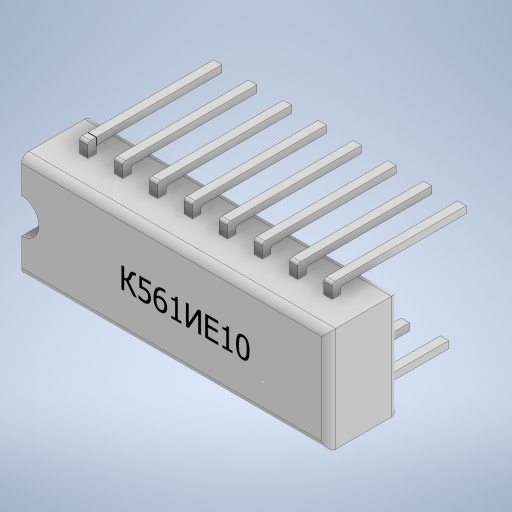
# Autodesk Inventor part: К561ИЕ10
Saved by Autodesk Inventor 2024 (Build 280153000, 153)
## iProperties
Created: 2023-12-20
Part Number: К561ИЕ10
Material: Generic
Document SubType Name: Sheet Metal
Designer: user
Density: 1 g/cm^3
Sheet Metal Rule: Default
Appearance: Default
Author: user
Autodesk Inventor part; units mm, degrees
ref_plane "YZ Plane" through (0, 0, 0) normal (1, 0, 0) x (0, 1, 0)
ref_plane "XZ Plane" through (0, 0, 0) normal (0, 1, 0) x (-1, 0, 0)
sketch "Sketch1" plane through (0, 0, 0) normal (0, 0, 1) x (1, 0, 0)
  line L0 (-17.2939, 5.4021) -> (4.7061, 5.4021)
  line L1 (4.7061, 5.4021) -> (4.7061, -2.0979)
  line L2 (4.7061, -2.0979) -> (-17.2939, -2.0979)
  line L3 (-17.2939, -2.0979) -> (-17.2939, 5.4021)
  line L4 (-17.2939, 5.4021) -> (-17.2939, 2.9021)
  line L5 (-17.2939, 2.9021) -> (-17.2939, 0.4021)
  line L6 (-17.2939, 0.4021) -> (-17.2939, -2.0979)
  arc A0 (-17.2939, 0.4021) -> (-17.2939, 2.9021) centre (-17.3071, 1.6521) ccw
  point P0 (0, 0)
  dimension "d0" = 22
  dimension "d1" = 7.5
  dimension "d2" = 2.5
  dimension "d3" = 2.5
  constraints: 14 end point, 2 parallel, 2 point on circle, 2 point on line, 1 centre point, 1 collinear, 1 horizontal, 1 perpendicular
  measures "d0" distance of L1.end L2.end
  measures "d1" distance of L0.end L1.end
  measures "d2" distance of L0.start L4.end
  measures "d3" distance of L4.end L5.end
extrude "Extrusion1" add sketch "Sketch1" along normal mid plane 5 contours L0 L1 L2 L3 A0
ref_plane "Work Plane1" through (0, 0, 0) normal (0, 0, 1) x (1, 0, 0)
sketch "Sketch2" plane through (0, 0, 0) normal (0, 0, 1) x (1, 0, 0)
  line L0 (4.7061, 5.4021) -> (-17.2939, 5.4021) projected
  line L1 (4.7061, 5.4021) -> (2.4561, 5.4021)
  line L2 (2.4561, 5.4021) -> (-0.0439, 5.4021)
  line L3 (-0.0439, 5.4021) -> (-2.5439, 5.4021)
  line L4 (-2.5439, 5.4021) -> (-5.0439, 5.4021)
  line L5 (-5.0439, 5.4021) -> (-7.5439, 5.4021)
  line L6 (-7.5439, 5.4021) -> (-10.0439, 5.4021)
  line L7 (-10.0439, 5.4021) -> (-12.5439, 5.4021)
  line L8 (-12.5439, 5.4021) -> (-15.0439, 5.4021)
  line L9 (-15.0439, 5.4021) -> (-17.2939, 5.4021)
  point P0 (0, 0)
  dimension "d6" = 2.25
  dimension "d7" = 2.5
  dimension "d8" = 2.5
  dimension "d9" = 2.5
  dimension "d10" = 2.5
  dimension "d11" = 2.5
  dimension "d12" = 2.5
  dimension "d13" = 2.5
  dimension "d14" = 2.25
  constraints: 18 end point, 1 horizontal, 9 other
  measures "d6" distance of L1.start L1.end
  measures "d7" distance of L1.end L2.end
  measures "d8" distance of L2.end L3.end
  measures "d9" distance of L3.end L4.end
  measures "d10" distance of L4.end L5.end
  measures "d11" distance of L5.end L6.end
  measures "d12" distance of L6.end L7.end
  measures "d13" distance of L7.end L8.end
  measures "d14" distance of L8.end L9.end
sketch "Sketch3" plane through (-17.2939, 5.4021, 2.5) normal (0, 1, 0) x (1, 0, 0)
  line L0 (20.1524, 2.9) -> (19.3524, 2.9)
  line L1 (19.3524, 2.9) -> (19.3524, 2.1)
  line L2 (19.3524, 2.1) -> (20.1524, 2.1)
  line L3 (20.1524, 2.1) -> (20.1524, 2.9)
  line L4 (20.1524, 2.9) -> (19.3524, 2.1) construction
  line L5 (19.3524, 2.9) -> (20.1524, 2.1) construction
  line L6 (17.6939, 2.9) -> (16.8939, 2.9)
  line L7 (16.8939, 2.9) -> (16.8939, 2.1)
  line L8 (16.8939, 2.1) -> (17.6939, 2.1)
  line L9 (17.6939, 2.1) -> (17.6939, 2.9)
  line L10 (17.6939, 2.9) -> (16.8939, 2.1) construction
  line L11 (16.8939, 2.9) -> (17.6939, 2.1) construction
  line L12 (15.1521, 2.1) -> (14.3521, 2.1)
  line L13 (14.3521, 2.1) -> (14.3521, 2.9)
  line L14 (14.3521, 2.9) -> (15.1521, 2.9)
  line L15 (15.1521, 2.9) -> (15.1521, 2.1)
  line L16 (15.1521, 2.1) -> (14.3521, 2.9) construction
  line L17 (14.3521, 2.1) -> (15.1521, 2.9) construction
  line L18 (12.6545, 2.1) -> (11.8545, 2.1)
  line L19 (11.8545, 2.1) -> (11.8545, 2.9)
  line L20 (11.8545, 2.9) -> (12.6545, 2.9)
  line L21 (12.6545, 2.9) -> (12.6545, 2.1)
  line L22 (12.6545, 2.1) -> (11.8545, 2.9) construction
  line L23 (11.8545, 2.1) -> (12.6545, 2.9) construction
  line L24 (10.1493, 2.9) -> (9.3493, 2.9)
  line L25 (9.3493, 2.9) -> (9.3493, 2.1)
  line L26 (9.3493, 2.1) -> (10.1493, 2.1)
  line L27 (10.1493, 2.1) -> (10.1493, 2.9)
  line L28 (10.1493, 2.9) -> (9.3493, 2.1) construction
  line L29 (9.3493, 2.9) -> (10.1493, 2.1) construction
  line L30 (7.6538, 2.1) -> (6.8538, 2.1)
  line L31 (6.8538, 2.1) -> (6.8538, 2.9)
  line L32 (6.8538, 2.9) -> (7.6538, 2.9)
  line L33 (7.6538, 2.9) -> (7.6538, 2.1)
  line L34 (7.6538, 2.1) -> (6.8538, 2.9) construction
  line L35 (6.8538, 2.1) -> (7.6538, 2.9) construction
  line L36 (5.1502, 2.1) -> (4.3502, 2.1)
  line L37 (4.3502, 2.1) -> (4.3502, 2.9)
  line L38 (4.3502, 2.9) -> (5.1502, 2.9)
  line L39 (5.1502, 2.9) -> (5.1502, 2.1)
  line L40 (5.1502, 2.1) -> (4.3502, 2.9) construction
  line L41 (4.3502, 2.1) -> (5.1502, 2.9) construction
  line L42 (2.649, 2.1) -> (1.849, 2.1)
  line L43 (1.849, 2.1) -> (1.849, 2.9)
  line L44 (1.849, 2.9) -> (2.649, 2.9)
  line L45 (2.649, 2.9) -> (2.649, 2.1)
  line L46 (2.649, 2.1) -> (1.849, 2.9) construction
  line L47 (1.849, 2.1) -> (2.649, 2.9) construction
  line L48 (20.0524, 2.8) -> (19.4524, 2.8)
  line L49 (19.4524, 2.8) -> (19.4524, 2.2)
  line L50 (19.4524, 2.2) -> (20.0524, 2.2)
  line L51 (20.0524, 2.2) -> (20.0524, 2.8)
  line L52 (20.0524, 2.8) -> (19.4524, 2.2) construction
  line L53 (19.4524, 2.8) -> (20.0524, 2.2) construction
  line L54 (17.5939, 2.8) -> (16.9939, 2.8)
  line L55 (16.9939, 2.8) -> (16.9939, 2.2)
  line L56 (16.9939, 2.2) -> (17.5939, 2.2)
  line L57 (17.5939, 2.2) -> (17.5939, 2.8)
  line L58 (17.5939, 2.8) -> (16.9939, 2.2) construction
  line L59 (16.9939, 2.8) -> (17.5939, 2.2) construction
  line L60 (15.0521, 2.8) -> (14.4521, 2.8)
  line L61 (14.4521, 2.8) -> (14.4521, 2.2)
  line L62 (14.4521, 2.2) -> (15.0521, 2.2)
  line L63 (15.0521, 2.2) -> (15.0521, 2.8)
  line L64 (15.0521, 2.8) -> (14.4521, 2.2) construction
  line L65 (14.4521, 2.8) -> (15.0521, 2.2) construction
  line L66 (12.5545, 2.8) -> (11.9545, 2.8)
  line L67 (11.9545, 2.8) -> (11.9545, 2.2)
  line L68 (11.9545, 2.2) -> (12.5545, 2.2)
  line L69 (12.5545, 2.2) -> (12.5545, 2.8)
  line L70 (12.5545, 2.8) -> (11.9545, 2.2) construction
  line L71 (11.9545, 2.8) -> (12.5545, 2.2) construction
  line L72 (9.4493, 2.8) -> (9.4493, 2.2)
  line L73 (10.0493, 2.2) -> (10.0493, 2.8)
  line L74 (10.0493, 2.8) -> (9.4493, 2.2) construction
  line L75 (9.4493, 2.8) -> (10.0493, 2.2) construction
  line L76 (10.0493, 2.8) -> (9.4493, 2.8)
  line L77 (9.4493, 2.2) -> (10.0493, 2.2)
  line L78 (6.9538, 2.8) -> (6.9538, 2.2)
  line L79 (7.5538, 2.2) -> (7.5538, 2.8)
  line L80 (7.5538, 2.8) -> (6.9538, 2.2) construction
  line L81 (6.9538, 2.8) -> (7.5538, 2.2) construction
  line L82 (7.5538, 2.8) -> (6.9538, 2.8)
  line L83 (6.9538, 2.2) -> (7.5538, 2.2)
  line L84 (4.4502, 2.8) -> (4.4502, 2.2)
  line L85 (5.0502, 2.2) -> (5.0502, 2.8)
  line L86 (5.0502, 2.8) -> (4.4502, 2.2) construction
  line L87 (4.4502, 2.8) -> (5.0502, 2.2) construction
  line L88 (5.0502, 2.8) -> (4.4502, 2.8)
  line L89 (4.4502, 2.2) -> (5.0502, 2.2)
  line L90 (1.949, 2.8) -> (1.949, 2.2)
  line L91 (2.549, 2.2) -> (2.549, 2.8)
  line L92 (2.549, 2.8) -> (1.949, 2.2) construction
  line L93 (1.949, 2.8) -> (2.549, 2.2) construction
  line L94 (2.549, 2.8) -> (1.949, 2.8)
  line L95 (1.949, 2.2) -> (2.549, 2.2)
  point P0 (17.2939, 2.5)
  dimension "d15" = 0.8
  dimension "d16" = 0.8
  dimension "d17" = 0.8
  dimension "d18" = 0.8
  dimension "d19" = 0.8
  dimension "d20" = 0.8
  dimension "d21" = 0.8
  dimension "d22" = 0.8
  dimension "d23" = 0.8
  dimension "d24" = 0.8
  dimension "d25" = 0.8
  dimension "d26" = 0.8
  dimension "d27" = 0.8
  dimension "d28" = 0.8
  dimension "d29" = 0.8
  dimension "d30" = 0.8
  dimension "d31" = 0.6
  dimension "d32" = 0.6
  dimension "d33" = 0.6
  dimension "d34" = 0.6
  dimension "d35" = 0.6
  dimension "d36" = 0.6
  dimension "d37" = 0.6
  dimension "d38" = 0.6
  dimension "d39" = 0.6
  dimension "d40" = 0.6
  dimension "d41" = 0.6
  dimension "d42" = 0.6
  dimension "d43" = 0.6
  dimension "d44" = 0.6
  dimension "d45" = 0.6
  dimension "d46" = 0.6
  constraints: 192 end point, 32 parallel, 16 horizontal, 16 perpendicular, 4 midpoint
  measures "d15" distance of L2.end L1.end
  measures "d16" distance of L1.end L0.end
  measures "d17" distance of L8.end L7.end
  measures "d18" distance of L7.end L6.end
  measures "d19" distance of L13.end L14.end
  measures "d20" distance of L12.end L13.end
  measures "d21" distance of L19.end L20.end
  measures "d22" distance of L18.end L19.end
  measures "d23" distance of L26.end L25.end
  measures "d24" distance of L25.end L24.end
  measures "d25" distance of L32.start L33.start
  measures "d26" distance of L30.end L32.start
  measures "d27" distance of L38.start L39.start
  measures "d28" distance of L36.end L38.start
  measures "d29" distance of L44.start L45.start
  measures "d30" distance of L42.end L44.start
  measures "d31" distance of L50.end L49.end
  measures "d32" distance of L49.end L48.end
  measures "d33" distance of L57.start L55.end
  measures "d34" distance of L55.end L55.start
  measures "d35" distance of L63.start L61.end
  measures "d36" distance of L61.end L61.start
  measures "d37" distance of L69.start L67.end
  measures "d38" distance of L67.end L67.start
  measures "d39" distance of L73.start L72.end
  measures "d40" distance of L72.end L72.start
  measures "d41" distance of L79.start L78.end
  measures "d42" distance of L78.end L78.start
  measures "d43" distance of L85.start L84.end
  measures "d44" distance of L84.end L84.start
  measures "d45" distance of L91.start L90.end
  measures "d46" distance of L90.end L90.start
extrude "Extrusion2" add sketch "Sketch3" along normal blind 1 contours L51 L50 L49 L48 | L57 L56 L55 L54 | L63 L62 L61 L60 | L69 L68 L67 L66 | L76 L73 L77 L72 | L82 L79 L83 L78 | L88 L85 L89 L84 | L94 L91 L95 L90
sketch "Sketch4" plane through (2.7586, 5.4021, -0.3) normal (0, 0, -1) x (-1, 0, 0)
  line L0 (0.6, 0) -> (0.6, 1) projected
  line L1 (0.6, 0.5) -> (0, 0.5)
  line L2 (0, 0) -> (0, 1) projected
  line L3 (2.4586, 0) -> (2.4586, 1) projected
  line L4 (2.4586, 0.5) -> (3.0586, 0.5)
  line L5 (3.0586, 0) -> (3.0586, 1) projected
  line L6 (5.0003, 0) -> (5.0003, 1) projected
  line L7 (5.0003, 0.5) -> (5.6003, 0.5)
  line L8 (5.6003, 0) -> (5.6003, 1) projected
  line L9 (7.4979, 0) -> (7.4979, 1) projected
  line L10 (7.4979, 0.5) -> (8.0979, 0.5)
  line L11 (8.0979, 0) -> (8.0979, 1) projected
  line L12 (10.0031, 0) -> (10.0031, 1) projected
  line L13 (10.0031, 0.5) -> (10.6031, 0.5)
  line L14 (10.6031, 0) -> (10.6031, 1) projected
  line L15 (12.4987, 0) -> (12.4987, 1) projected
  line L16 (12.4987, 0.5) -> (13.0987, 0.5)
  line L17 (13.0987, 0) -> (13.0987, 1) projected
  line L18 (15.0022, 0) -> (15.0022, 1) projected
  line L19 (15.0022, 0.5) -> (15.6022, 0.5)
  line L20 (15.6022, 0) -> (15.6022, 1) projected
  line L21 (17.5034, 0) -> (17.5034, 1) projected
  line L22 (17.5034, 0.5) -> (18.1034, 0.5)
  line L23 (18.1034, 0) -> (18.1034, 1) projected
  line L24 (17.5034, 0.5) -> (17.5034, 1)
  line L25 (17.5034, 1) -> (18.1034, 1)
  line L26 (18.1034, 1) -> (18.1034, 0.5)
  point P0 (2.7586, -5.4021)
  constraints: 22 end point, 16 midpoint, 2 perpendicular
sketch "Sketch5" plane through (2.7586, 5.4021, -0.3) normal (0, 0, -1) x (-1, 0, 0)
  line L0 (0, 0) -> (0, 1) projected
  line L1 (0, 0.5) -> (0, 1)
  line L2 (0.6, 1) -> (0, 1) projected
  line L3 (0, 1) -> (0.6, 1)
  line L4 (0.6, 1) -> (0.6, 0.5)
  line L5 (0.6, 0.5) -> (0, 0.5)
  point P0 (2.7586, -5.4021)
  constraints: 8 end point, 3 perpendicular, 1 collinear, 1 midpoint
sketch "Sketch6" plane through (0.3, 5.4021, -0.3) normal (0, 0, -1) x (-1, 0, 0)
  line L0 (0, 0.5) -> (0, 1)
  line L1 (0, 1) -> (0.6, 1)
  line L2 (0.6, 1) -> (0.6, 0.5)
  line L3 (0.6, 0.5) -> (0, 0.5)
  point P0 (2.7586, -5.4021)
  constraints: 8 end point, 3 perpendicular
sketch "Sketch7" plane through (-2.2417, 5.4021, -0.3) normal (0, 0, -1) x (-1, 0, 0)
  line L0 (0, 0.5) -> (0, 1)
  line L1 (0, 1) -> (0.6, 1)
  line L2 (0.6, 1) -> (0.6, 0.5)
  line L3 (0.6, 0.5) -> (0, 0.5)
  point P0 (2.7586, -5.4021)
  constraints: 8 end point, 3 perpendicular
sketch "Sketch8" plane through (-4.7394, 5.4021, -0.3) normal (0, 0, -1) x (-1, 0, 0)
  line L0 (0, 0.5) -> (0, 1)
  line L1 (0, 1) -> (0.6, 1)
  line L2 (0.6, 1) -> (0.6, 0.5)
  line L3 (0.6, 0.5) -> (0, 0.5)
  point P0 (2.7586, -5.4021)
  constraints: 8 end point, 3 perpendicular
sketch "Sketch9" plane through (-7.2446, 5.4021, -0.3) normal (0, 0, -1) x (-1, 0, 0)
  line L0 (0, 0.5) -> (0, 1)
  line L1 (0, 1) -> (0.6, 1)
  line L2 (0.6, 1) -> (0.6, 0.5)
  line L3 (0.6, 0.5) -> (0, 0.5)
  point P0 (2.7586, -5.4021)
  constraints: 8 end point, 3 perpendicular
sketch "Sketch10" plane through (-9.7401, 5.4021, -0.3) normal (0, 0, -1) x (-1, 0, 0)
  line L0 (0, 0.5) -> (0, 1)
  line L1 (0, 1) -> (0.6, 1)
  line L2 (0.6, 1) -> (0.6, 0.5)
  line L3 (0.6, 0.5) -> (0, 0.5)
  point P0 (2.7586, -5.4021)
  constraints: 8 end point, 3 perpendicular
sketch "Sketch11" plane through (-12.2436, 5.4021, -0.3) normal (0, 0, -1) x (-1, 0, 0)
  line L0 (0, 0.5) -> (0, 1)
  line L1 (0, 1) -> (0.6, 1)
  line L2 (0.6, 1) -> (0.6, 0.5)
  line L3 (0.6, 0.5) -> (0, 0.5)
  point P0 (2.7586, -5.4021)
  constraints: 8 end point, 3 perpendicular
sketch "Sketch12" plane through (-14.7449, 5.4021, -0.3) normal (0, 0, -1) x (-1, 0, 0)
  line L0 (0, 0.5) -> (0, 1)
  line L1 (0, 1) -> (0.6, 1)
  line L2 (0.6, 1) -> (0.6, 0.5)
  line L3 (0.6, 0.5) -> (0, 0.5)
  point P0 (2.7586, -5.4021)
  constraints: 8 end point, 3 perpendicular
extrude "Extrusion3" add sketch "Sketch5" along normal blind 9
extrude "Extrusion4" add sketch "Sketch6" along normal blind 9
extrude "Extrusion5" add sketch "Sketch7" along normal blind 9
extrude "Extrusion6" add sketch "Sketch8" along normal blind 9
extrude "Extrusion7" add sketch "Sketch9" along normal blind 9
extrude "Extrusion8" add sketch "Sketch10" along normal blind 9
extrude "Extrusion9" add sketch "Sketch11" along normal blind 9
extrude "Extrusion10" add sketch "Sketch4" along normal blind 9
fillet "Fillet1" radius 0.2 16 edges at (2.4586, 6.4021, 0.3) (2.4586, 5.9021, -0.3) (0, 6.4021, 0.3) (0, 5.9021, -0.3) (-2.5417, 6.4021, 0.3) (-2.5417, 5.9021, -0.3) (-5.0394, 6.4021, 0.3) (-5.0394, 5.9021, -0.3) (-7.5446, 6.4021, 0.3) (-7.5446, 5.9021, -0.3) (-10.0401, 6.4021, 0.3) (-10.0401, 5.9021, -0.3) (-12.5436, 6.4021, 0.3) (-12.5436, 5.9021, -0.3) (-15.0449, 6.4021, 0.3) (-15.0449, 5.9021, -0.3)
fillet "Fillet2" radius 0.5 3 edges at (-6.2939, 5.4021, 2.5) (-6.2939, -2.0979, 2.5) (4.7061, 1.6521, 2.5)
fillet "Fillet3" radius 0.5 3 edges at (-6.2939, 5.4021, -2.5) (4.7061, 1.6521, -2.5) (-6.2939, -2.0979, -2.5)
sketch "Sketch13" plane through (-17.2939, -2.0979, 2) normal (0, -1, 0) x (1, 0, 0)
  line L0 (0, -4.5) -> (0, 0.5) projected
  line L1 (0, -2) -> (2.25, -2)
  line L2 (2.25, -2) -> (4.75, -2)
  line L3 (4.75, -2) -> (7.25, -2)
  line L4 (7.25, -2) -> (9.75, -2)
  line L5 (9.75, -2) -> (12.25, -2)
  line L6 (12.25, -2) -> (14.75, -2)
  line L7 (14.75, -2) -> (17.25, -2)
  line L8 (17.25, -2) -> (19.75, -2)
  line L9 (19.75, -2) -> (22, -2)
  line L10 (3.2, -1.7) -> (3.8, -1.7)
  line L11 (3.8, -1.7) -> (3.8, -2.3)
  line L12 (3.8, -2.3) -> (3.2, -2.3)
  line L13 (3.2, -2.3) -> (3.2, -1.7)
  line L14 (3.2, -1.7) -> (3.8, -2.3) construction
  line L15 (3.8, -1.7) -> (3.2, -2.3) construction
  line L16 (5.7, -1.7) -> (6.3, -1.7)
  line L17 (6.3, -1.7) -> (6.3, -2.3)
  line L18 (6.3, -2.3) -> (5.7, -2.3)
  line L19 (5.7, -2.3) -> (5.7, -1.7)
  line L20 (5.7, -1.7) -> (6.3, -2.3) construction
  line L21 (6.3, -1.7) -> (5.7, -2.3) construction
  line L22 (8.2, -1.7) -> (8.8, -1.7)
  line L23 (8.8, -1.7) -> (8.8, -2.3)
  line L24 (8.8, -2.3) -> (8.2, -2.3)
  line L25 (8.2, -2.3) -> (8.2, -1.7)
  line L26 (8.2, -1.7) -> (8.8, -2.3) construction
  line L27 (8.8, -1.7) -> (8.2, -2.3) construction
  line L28 (10.7, -1.7) -> (11.3, -1.7)
  line L29 (11.3, -1.7) -> (11.3, -2.3)
  line L30 (11.3, -2.3) -> (10.7, -2.3)
  line L31 (10.7, -2.3) -> (10.7, -1.7)
  line L32 (10.7, -1.7) -> (11.3, -2.3) construction
  line L33 (11.3, -1.7) -> (10.7, -2.3) construction
  line L34 (13.2, -1.7) -> (13.8, -1.7)
  line L35 (13.8, -1.7) -> (13.8, -2.3)
  line L36 (13.8, -2.3) -> (13.2, -2.3)
  line L37 (13.2, -2.3) -> (13.2, -1.7)
  line L38 (13.2, -1.7) -> (13.8, -2.3) construction
  line L39 (13.8, -1.7) -> (13.2, -2.3) construction
  line L40 (15.7, -1.7) -> (16.3, -1.7)
  line L41 (16.3, -1.7) -> (16.3, -2.3)
  line L42 (16.3, -2.3) -> (15.7, -2.3)
  line L43 (15.7, -2.3) -> (15.7, -1.7)
  line L44 (15.7, -1.7) -> (16.3, -2.3) construction
  line L45 (16.3, -1.7) -> (15.7, -2.3) construction
  line L46 (18.8, -1.7) -> (18.8, -2.3)
  line L47 (18.8, -2.3) -> (18.2, -2.3)
  line L48 (18.2, -2.3) -> (18.2, -1.7)
  line L49 (18.2, -1.7) -> (18.8, -1.7)
  line L50 (18.8, -1.7) -> (18.2, -2.3) construction
  line L51 (18.2, -1.7) -> (18.8, -2.3) construction
  point P0 (17.2939, -2)
  point P1 (3.5, -2)
  point P2 (6, -2)
  point P3 (8.5, -2)
  point P4 (11, -2)
  point P5 (13.5, -2)
  point P6 (16, -2)
  point P7 (18.5, -2)
  point P8 (15.7, -2)
  point P9 (16.3, -2)
  dimension "d76" = 2.25
  dimension "d77" = 2.5
  dimension "d78" = 2.5
  dimension "d79" = 2.5
  dimension "d80" = 2.5
  dimension "d81" = 2.5
  dimension "d82" = 2.5
  dimension "d83" = 2.5
  dimension "d84" = 2.25
  dimension "d87" = 0.6
  dimension "d88" = 0.6
  dimension "d89" = 0.6
  dimension "d90" = 0.6
  dimension "d91" = 0.6
  dimension "d92" = 0.6
  dimension "d93" = 0.6
  dimension "d94" = 0.6
  dimension "d95" = 0.6
  dimension "d96" = 0.6
  dimension "d97" = 0.6
  dimension "d98" = 0.6
  dimension "d99" = 0.6
  dimension "d100" = 0.6
  constraints: 102 end point, 22 midpoint, 14 parallel, 8 horizontal, 8 point on line, 7 perpendicular
  measures "d76" distance of L1.start L1.end
  measures "d77" distance of L1.end L2.end
  measures "d78" distance of L2.end L3.end
  measures "d79" distance of L3.end L4.end
  measures "d80" distance of L4.end L5.end
  measures "d81" distance of L5.end L6.end
  measures "d82" distance of L6.end L7.end
  measures "d83" distance of L7.end L8.end
  measures "d84" distance of L8.end L9.end
  measures "d87" distance of L11.end L12.end
  measures "d88" distance of L10.end L11.end
  measures "d89" distance of L17.end L18.end
  measures "d90" distance of L17.start L17.end
  measures "d91" distance of L23.end L24.end
  measures "d92" distance of L23.start L23.end
  measures "d93" distance of L29.end L30.end
  measures "d94" distance of L29.start L29.end
  measures "d95" distance of L35.end L36.end
  measures "d96" distance of L35.start L35.end
  measures "d97" distance of L41.end L42.end
  measures "d98" distance of L41.start L41.end
  measures "d99" distance of L46.end L48.start
  measures "d100" distance of L46.start L46.end
extrude "Extrusion11" add sketch "Sketch13" along normal blind 1 contours L13 L10 L11 L2 | L2 L11 L12 L13 | L48 L49 L46 L8 | L8 L46 L47 L48 | L43 L40 L41 L7 | L37 L34 L35 L6 | L6 L35 L36 L37 | L31 L28 L29 L5 | L5 L29 L30 L31 | L25 L22 L23 L4 | L4 L23 L24 L25 | L19 L16 L17 L3 | L3 L17 L18 L19
sketch "Sketch14" plane through (-13.4939, -2.0979, -0.3) normal (0, 0, -1) x (-1, 0, 0)
  line L0 (0.6, 0) -> (0.6, -1) projected
  line L1 (0.6, -0.5) -> (0, -0.5)
  line L2 (0, 0) -> (0, -1) projected
  line L3 (0, -1) -> (0.6, -1) projected
  line L4 (0, -1) -> (0.6, -1)
  line L5 (0.6, 0) -> (0.6, -1) projected
  line L6 (0.6, -0.5) -> (0.6, -1)
  line L7 (0, -1) -> (0, -0.5)
  point P0 (-13.4939, 2.0979)
  constraints: 8 end point, 2 collinear, 2 midpoint, 1 horizontal
sketch "Sketch15" plane through (-10.9939, -2.0979, -0.3) normal (0, 0, -1) x (-1, 0, 0)
  line L0 (0.6, -0.5) -> (0, -0.5)
  line L1 (0, -1) -> (0.6, -1)
  line L2 (0.6, -0.5) -> (0.6, -1)
  line L3 (0, -1) -> (0, -0.5)
  point P0 (-13.4939, 2.0979)
  constraints: 8 end point, 1 horizontal
extrude "Extrusion12" add sketch "Sketch15" along normal blind 9
extrude "Extrusion13" add sketch "Sketch14" along normal blind 9
sketch "Sketch16" plane through (-8.4939, -2.0979, -0.3) normal (0, 0, -1) x (-1, 0, 0)
  line L0 (0.6, -0.5) -> (0, -0.5)
  line L1 (0, -1) -> (0.6, -1)
  line L2 (0.6, -0.5) -> (0.6, -1)
  line L3 (0, -1) -> (0, -0.5)
  point P0 (-13.4939, 2.0979)
  constraints: 8 end point, 1 horizontal
sketch "Sketch17" plane through (-3.4939, -2.0979, -0.3) normal (0, 0, -1) x (-1, 0, 0)
  line L0 (0.6, -0.5) -> (0, -0.5)
  line L1 (0, -1) -> (0.6, -1)
  line L2 (0.6, -0.5) -> (0.6, -1)
  line L3 (0, -1) -> (0, -0.5)
  point P0 (-13.4939, 2.0979)
  constraints: 8 end point, 1 horizontal
sketch "Sketch18" plane through (-5.9939, -2.0979, -0.3) normal (0, 0, -1) x (-1, 0, 0)
  line L0 (0.6, -0.5) -> (0, -0.5)
  line L1 (0, -1) -> (0.6, -1)
  line L2 (0.6, -0.5) -> (0.6, -1)
  line L3 (0, -1) -> (0, -0.5)
  point P0 (-13.4939, 2.0979)
  constraints: 8 end point, 1 horizontal
sketch "Sketch19" plane through (-0.9939, -2.0979, 0) normal (0, 0, -1) x (-1, 0, 0)
  line L0 (0.6, -0.5) -> (0, -0.5)
  line L1 (0, -1) -> (0.6, -1)
  line L2 (0.6, -0.5) -> (0.6, -1)
  line L3 (0, -1) -> (0, -0.5)
  point P0 (-13.4939, 2.0979)
  constraints: 8 end point, 1 horizontal
sketch "Sketch20" plane through (1.5061, -2.0979, -0.3) normal (0, 0, -1) x (-1, 0, 0)
  line L0 (0.6, -0.5) -> (0, -0.5)
  line L1 (0, -1) -> (0.6, -1)
  line L2 (0.6, -0.5) -> (0.6, -1)
  line L3 (0, -1) -> (0, -0.5)
  point P0 (-13.4939, 2.0979)
  constraints: 8 end point, 1 horizontal
extrude "Extrusion14" add sketch "Sketch16" along normal blind 9
extrude "Extrusion15" add sketch "Sketch18" along normal blind 9
extrude "Extrusion16" add sketch "Sketch17" along normal blind 9
extrude "Extrusion17" add sketch "Sketch19" along normal blind 9
extrude "Extrusion18" add sketch "Sketch20" along normal blind 9
fillet "Fillet4" radius 0.5 14 edges at (-13.7939, -3.0979, 0.3) (-13.7939, -2.5979, -0.3) (-11.2939, -3.0979, 0.3) (-11.2939, -2.5979, -0.3) (-8.7939, -3.0979, 0.3) (-8.7939, -2.5979, -0.3) (-6.2939, -3.0979, 0.3) (-6.2939, -2.5979, -0.3) (-3.7939, -3.0979, 0.3) (-3.7939, -2.5979, -0.3) (-1.2939, -3.0979, 0.3) (-1.2939, -2.5979, 0) (1.2061, -3.0979, 0.3) (1.2061, -2.5979, -0.3)
sketch "Sketch21" plane through (0, 0, 2.5) normal (0, 0, 1) x (1, 0, 0)
  line L0 (-10.2931, 2.1964) -> (-0.8823, 2.1964) construction
  line L1 (-0.8823, 2.1964) -> (-0.8823, 0.6344) construction
  line L2 (-0.8823, 0.6344) -> (-10.2931, 0.6344) construction
  line L3 (-10.2931, 0.6344) -> (-10.2931, 2.1964) construction
  point P0 (0, 0)
  constraints: 2 other
equation "\"BendRadius\" = Thickness"
equation "\"BendReliefWidth\" = Thickness"
equation "\"BendReliefDepth\" = 0.5 * Thickness"
equation "\"CornerReliefSize\" = 4 * Thickness"
equation "\"MinimumRemnant\" = 2 * Thickness"
equation "\"TransitionRadius\" = BendRadius"
equation "\"JacobiRadiusSize\" = BendRadius"
equation "\"GapSize\" = Thickness"
equation "\"Thickness\" = 3.048"
body "Solid1"
